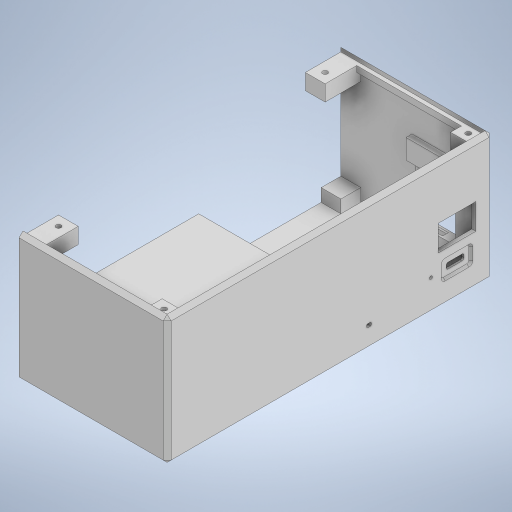
# Autodesk Inventor part: base
Saved by Autodesk Inventor 2024.2 (Build 282272000, 272)
## iProperties
Created: 2024-05-15
Part Number: base
Material: Générique
Document SubType Name: Modeling
Designer: michgae
Density: 1 g/cm^3
Appearance: Par défaut
Author: michgae
Autodesk Inventor part; units mm, degrees
ref_plane "YZ Plane" through (0, 0, 0) normal (1, 0, 0) x (0, 1, 0)
ref_plane "XZ Plane" through (0, 0, 0) normal (0, 1, 0) x (-1, 0, 0)
ref_plane "XY Plane" through (0, 0, 0) normal (0, 0, 1) x (1, 0, 0)
sketch "Esquisse1" plane through (0, 0, 0) normal (0, 0, 1) x (1, 0, 0)
  line L0 (37.5, -32.5) -> (-37.5, -32.5)
  line L1 (-37.5, -32.5) -> (-37.5, 32.5)
  line L2 (-37.5, 32.5) -> (37.5, 32.5)
  line L3 (37.5, 32.5) -> (37.5, -32.5)
  line L4 (0, -45.5) -> (0, 45.5) projected
  line L5 (-52.5, 0) -> (52.5, 0) projected
  line L6 (-37.5, -30.5) -> (35.5, -30.5)
  line L7 (35.5, -30.5) -> (35.5, 32.5)
  point P0 (0, 0)
  dimension "d0" = 75
  dimension "d1" = 65
  dimension "d2" = 32.5
  dimension "d3" = 2
  dimension "d4" = 2
  constraints: 12 end point, 2 horizontal, 2 parallel, 2 perpendicular, 2 point on line, 1 other
  measures "d0" distance of L2.end L1.end
  measures "d1" distance of L1.end L0.end
  measures "d2" distance between parallel lines of L5 L0
  measures "d3" distance between parallel lines of L3 L7
  measures "d4" distance between parallel lines of L0 L6
extrude "Extrusion1" add sketch "Esquisse1" along normal blind 2
extrude "Extrusion2" add sketch "Esquisse1" against normal blind 161 contours L0 L4 L6 L7 L5 L3 | L0 L1 L6 L4 | L5 L7 L2 L3
sketch "Esquisse4" plane through (0, 0, -161) normal (0, 0, -1) x (-1, 0, 0)
  line L0 (37.5, 32.5) -> (37.5, -32.5) projected
  line L1 (-37.5, -32.5) -> (37.5, -32.5)
  line L2 (37.5, -32.5) -> (37.5, 32.5)
  line L3 (37.5, 32.5) -> (-37.5, 32.5)
  line L4 (-37.5, 32.5) -> (-37.5, -32.5)
  point P0 (0, 0)
  constraints: 8 end point, 2 parallel, 1 horizontal, 1 perpendicular
extrude "Extrusion5" add sketch "Esquisse4" along normal blind 2
sketch "Esquisse7" plane through (-37.5, -30.5, 0) normal (0, 1, 0) x (1, 0, 0)
  circle A0 centre (69.5, 152.5) radius 1
  line L0 (73, 0) -> (73, 161) projected
  line L1 (0, 161) -> (73, 161) projected
  circle A1 centre (68.5, 9.5) radius 1
  line L2 (73, 0) -> (0, 0) projected
  line L3 (73, 161) -> (63, 161)
  line L4 (63, 161) -> (63, 146)
  line L5 (63, 146) -> (73, 146)
  line L6 (73, 146) -> (73, 161)
  line L7 (73, 0) -> (63, 0)
  line L8 (63, 0) -> (63, 15)
  line L9 (63, 15) -> (73, 15)
  line L10 (73, 15) -> (73, 0)
  point P0 (37.5, 0)
  point P1 (63, 0)
  dimension "d32" = 2
  dimension "d33" = 3.5
  dimension "d34" = 8.5
  dimension "d35" = 2
  dimension "d36" = 4.5
  dimension "d37" = 9.5
  dimension "d38" = 10
  dimension "d39" = 15
  dimension "d40" = 15
  dimension "d41" = 10
  constraints: 16 end point, 4 parallel, 2 centre point, 2 horizontal, 2 perpendicular
  measures "d32" diameter of A0
  measures "d33" distance from line of L0 A0.centre
  measures "d34" distance from line of L1 A0.centre
  measures "d35" diameter of A1
  measures "d36" distance from line of L0 A1.centre
  measures "d37" distance from line of L2 A1.centre
  measures "d38" distance of L5.end L4.end
  measures "d39" distance of L4.end L3.end
  measures "d40" distance of L7.end L8.end
  measures "d41" distance of L8.end L9.end
extrude "Extrusion7" add sketch "Esquisse7" along normal blind 6.5
sketch "Esquisse8" plane through (35.5, 32.5, -161) normal (-1, 0, 0) x (0, 0, 1)
  line L0 (12.7, -50.3) -> (19.7, -50.3)
  line L1 (20.7, -49.3) -> (20.7, -48.3)
  line L2 (19.7, -47.3) -> (12.7, -47.3)
  line L3 (11.7, -48.3) -> (11.7, -49.3)
  line L4 (0, -56.5) -> (15, -56.5) projected
  line L5 (10.2, -44.8) -> (22.2, -44.8)
  line L6 (23.2, -45.8) -> (23.2, -51.8)
  line L7 (22.2, -52.8) -> (10.2, -52.8)
  line L8 (9.2, -51.8) -> (9.2, -45.8)
  line L9 (0, -63) -> (0, 0) projected
  arc A0 (12.7, -47.3) -> (11.7, -48.3) centre (12.7, -48.3) ccw
  arc A1 (11.7, -49.3) -> (12.7, -50.3) centre (12.7, -49.3) ccw
  arc A2 (19.7, -50.3) -> (20.7, -49.3) centre (19.7, -49.3) ccw
  arc A3 (20.7, -48.3) -> (19.7, -47.3) centre (19.7, -48.3) ccw
  arc A4 (10.2, -44.8) -> (9.2, -45.8) centre (10.2, -45.8) ccw
  arc A5 (23.2, -45.8) -> (22.2, -44.8) centre (22.2, -45.8) ccw
  arc A6 (22.2, -52.8) -> (23.2, -51.8) centre (22.2, -51.8) ccw
  arc A7 (9.2, -51.8) -> (10.2, -52.8) centre (10.2, -51.8) ccw
  circle A8 centre (29.45, -48.8) radius 0.75
  circle A9 centre (60.8, -53.85) radius 1.25
  line L10 (59.9, -52.9825) -> (61.7, -52.9825)
  line L11 (59.9, -54.7175) -> (61.7, -54.7175)
  line L12 (6.7, -39.8) -> (25.7, -39.8)
  line L13 (25.7, -39.8) -> (25.7, -26.8)
  line L14 (25.7, -26.8) -> (6.7, -26.8)
  line L15 (6.7, -26.8) -> (6.7, -39.8)
  point P0 (161, -32.5)
  point P1 (11.7, -50.3)
  point P2 (20.7, -47.3)
  point P3 (11.7, -47.3)
  point P4 (9.2, -44.8)
  point P5 (23.2, -52.8)
  point P6 (23.2, -44.8)
  point P7 (16.2, -52.8)
  dimension "d44" = 6.2
  dimension "d45" = 3
  dimension "d46" = 8
  dimension "d47" = 14
  dimension "d48" = 9
  dimension "d49" = 2.5
  dimension "d50" = 11.7
  dimension "d52" = 1
  dimension "d57" = 9.2
  dimension "d58" = 1.5
  dimension "d59" = 6.25
  dimension "d60" = 4
  dimension "d63" = 2.5
  dimension "d64" = 60.8
  dimension "d65" = 2.65
  dimension "d68" = 1.8
  dimension "d69" = 1.8
  dimension "d70" = 19
  dimension "d71" = 13
  dimension "d72" = 2.5
  dimension "d73" = 5
  constraints: 28 end point, 20 point on circle, 16 tangent, 12 point on line, 10 centre point, 7 equal radius, 6 parallel, 5 horizontal, 3 perpendicular, 1 midpoint
  measures "d44" distance between parallel lines of L0 L4
  measures "d45" distance of point (11.7, -47.3) point (11.7, -50.3)
  measures "d46" distance of point (23.2, -44.8) point (23.2, -52.8)
  measures "d47" distance of point (9.2, -44.8) point (23.2, -44.8)
  measures "d48" distance of point (20.7, -47.3) point (11.7, -47.3)
  measures "d49" distance from line of point (16.2, -52.8) L0
  measures "d50" distance between parallel lines of L3 L9
  measures "d52" radius of A0
  measures "d57" distance between parallel lines of L9 L8
  measures "d58" diameter of A8
  measures "d59" distance from line of L6 A8.centre
  measures "d60" distance from line of L7 A8.centre
  measures "d63" diameter of A9
  measures "d64" distance from line of L9 A9.centre
  measures "d65" distance from line of L4 A9.centre
  measures "d68" distance of L10.start L10.end
  measures "d69" distance of L11.start L11.end
  measures "d70" distance of L14.end L13.end
  measures "d71" distance of L13.end L12.end
  measures "d72" distance between parallel lines of L6 L13
  measures "d73" distance between parallel lines of L12 L5
extrude "Extrusion8" cut sketch "Esquisse8" against normal through all contours A1 L3 A0 L2 A3 L1 A2 L0 | L5 A5 L6 A6 L7 A7 L8 A4
extrude "Extrusion9" add sketch "Esquisse8" against normal blind 1 contours L5 A5 L6 A6 L7 A7 L8 A4
extrude "Extrusion10" cut sketch "Esquisse8" against normal through all contours A8
extrude "Extrusion11" cut sketch "Esquisse8" against normal through all contours A9 L11 L10
extrude "Extrusion12" cut sketch "Esquisse8" against normal through all contours L15 L14 L13 L12
sketch "Esquisse9" plane through (0, 0, -161) normal (0, 0, 1) x (1, 0, 0)
  line L0 (0.5, -22.5) -> (20.5, -22.5)
  line L1 (20.5, -22.5) -> (20.5, 7.5)
  line L2 (20.5, 7.5) -> (0.5, 7.5)
  line L3 (0.5, 7.5) -> (0.5, -22.5)
  line L4 (35.5, -24) -> (35.5, 32.5) projected
  line L5 (-37.5, -30.5) -> (25.5, -30.5) projected
  line L6 (-1.5, 12.5) -> (22.5, 12.5)
  line L7 (22.5, 12.5) -> (22.5, 2.5)
  line L8 (22.5, 2.5) -> (-1.5, 2.5)
  line L9 (-1.5, 2.5) -> (-1.5, 12.5)
  circle A0 centre (10.5, 5) radius 1.25
  line L10 (23, -22.5) -> (-2, -22.5)
  line L11 (-2, -22.5) -> (-2, -27.5)
  line L12 (-2, -27.5) -> (23, -27.5)
  line L13 (23, -27.5) -> (23, -22.5)
  line L14 (-37.5, 32.5) -> (-27.5, 32.5)
  line L15 (-27.5, 32.5) -> (-27.5, 22.5)
  line L16 (-27.5, 22.5) -> (-37.5, 22.5)
  line L17 (-37.5, 22.5) -> (-37.5, 32.5)
  line L18 (-37.5, -30.5) -> (-27.5, -30.5)
  line L19 (-27.5, -30.5) -> (-27.5, -24)
  line L20 (-27.5, -24) -> (-37.5, -24)
  line L21 (-37.5, -24) -> (-37.5, -30.5)
  point P0 (0, 0)
  point P1 (22.5, 7.5)
  point P2 (-1.5, 7.5)
  point P3 (23, -25)
  dimension "d77" = 35
  dimension "d78" = 20
  dimension "d79" = 8
  dimension "d80" = 30
  dimension "d81" = 2
  dimension "d82" = 2
  dimension "d83" = 5
  dimension "d84" = 10
  dimension "d85" = 2.5
  dimension "d86" = 2.5
  dimension "d87" = 10
  dimension "d88" = 25
  dimension "d89" = 2.5
  dimension "d90" = 5
  dimension "d104" = 10
  dimension "d105" = 10
  dimension "d113" = 10
  dimension "d114" = 6.5
  constraints: 40 end point, 10 parallel, 5 horizontal, 5 perpendicular, 3 midpoint, 1 centre point, 1 collinear
  measures "d77" distance between parallel lines of L4 L3
  measures "d78" distance of L1.end L2.end
  measures "d79" distance between parallel lines of L0 L5
  measures "d80" distance of L2.end L0.start
  measures "d81" distance from line of point (22.5, 7.5) L1
  measures "d82" distance from line of L3 point (-1.5, 7.5)
  measures "d83" distance between parallel lines of L2 L6
  measures "d84" distance between parallel lines of L6 L8
  measures "d85" diameter of A0
  measures "d86" distance from line of L2 A0.centre
  measures "d87" distance from line of L1 A0.centre
  measures "d88" distance of L12.end L11.end
  measures "d89" distance from line of L1 point (23, -25)
  measures "d90" distance of L10.end L11.end
  measures "d104" distance of L15.end L16.end
  measures "d105" distance of L14.end L15.end
  measures "d113" distance of L20.end L19.end
  measures "d114" distance of L19.end L18.end
extrude "Extrusion13" cut sketch "Esquisse9" against normal blind 10 contours L3 L8 L1 L0 | L3 L2 L1 L8 | A0
extrude "Extrusion14" add sketch "Esquisse9" along normal blind 3 contours L0 L10 L13 L12 L11 | L8 L9 L6 L7 L1 L2 L3 | L3 L2 L1 L8
sketch "Esquisse10" plane through (0.5, -22.5, -163) normal (0, 1, 0) x (1, 0, 0)
  line L0 (15, -1.5) -> (5, -1.5)
  line L1 (5, -1.5) -> (5, -3.5)
  line L2 (5, -3.5) -> (15, -3.5)
  line L3 (15, -3.5) -> (15, -1.5)
  line L4 (0, 0) -> (20, 0) projected
  line L5 (20, -2) -> (20, 0) projected
  point P0 (-0.5, -163)
  dimension "d95" = 10
  dimension "d96" = 2
  dimension "d97" = 1.5
  dimension "d98" = 5
  constraints: 8 end point, 2 parallel, 1 horizontal, 1 perpendicular
  measures "d95" distance of L1.end L2.end
  measures "d96" distance of L0.end L1.end
  measures "d97" distance between parallel lines of L4 L0
  measures "d98" distance between parallel lines of L5 L3
extrude "Extrusion15" cut sketch "Esquisse10" against normal blind 3
chamfer "Chanfrein1" distance 0.5 angle 45 4 edges at (15.5, -22.5, -160.5) (10.5, -22.5, -159.5) (10.5, -22.5, -161.5) (5.5, -22.5, -160.5)
extrude "Extrusion16" add sketch "Esquisse9" along normal blind 18 contours L14 L15 L16 L17
extrude "Extrusion18" add sketch "Esquisse9" along normal blind 10 contours L21 L20 L19 L5
sketch "Esquisse12" plane through (0, 0, 0) normal (0, 0, -1) x (-1, 0, 0)
  line L0 (-25.5, -30.5) -> (37.5, -30.5) projected
  line L1 (37.5, -30.5) -> (27.5, -30.5)
  line L2 (27.5, -30.5) -> (27.5, -24)
  line L3 (27.5, -24) -> (37.5, -24)
  line L4 (37.5, -24) -> (37.5, -30.5)
  line L5 (37.5, 32.5) -> (37.5, -32.5) projected
  line L6 (37.5, 32.5) -> (27.5, 32.5)
  line L7 (27.5, 32.5) -> (27.5, 22.5)
  line L8 (27.5, 22.5) -> (37.5, 22.5)
  line L9 (37.5, 22.5) -> (37.5, 32.5)
  point P0 (0, 0)
  dimension "d120" = 10
  dimension "d121" = 6.5
  dimension "d122" = 10
  dimension "d123" = 10
  constraints: 16 end point, 4 parallel, 2 horizontal, 2 perpendicular
  measures "d120" distance of L2.end L3.end
  measures "d121" distance of L1.end L2.end
  measures "d122" distance of L8.end L7.end
  measures "d123" distance of L7.end L6.end
extrude "Extrusion19" add sketch "Esquisse12" along normal blind 18 contours L5 L8 L7 L6
extrude "Extrusion20" add sketch "Esquisse12" along normal blind 10 contours L2 L3 L4 L0
sketch "Esquisse11" plane through (-37.5, -32.5, 2) normal (-1, 0, 0) x (0, 0, 1)
  circle A0 centre (-160, 60) radius 1.25
  line L0 (-145, 65) -> (-165, 65) projected
  line L1 (-165, 0) -> (-165, 65) projected
  circle A1 centre (-160, 5) radius 1.25
  line L2 (-165, 0) -> (0, 0) projected
  circle A2 centre (-5, 60) radius 1.25
  circle A3 centre (-5, 5) radius 1.25
  point P0 (-2, 32.5)
  dimension "d108" = 2.5
  dimension "d109" = 5
  dimension "d110" = 5
  dimension "d117" = 2.5
  dimension "d118" = 5
  dimension "d119" = 5
  dimension "d130" = 155
  constraints: 4 centre point, 1 horizontal, 4 other
  measures "d108" diameter of A0
  measures "d109" distance from line of L0 A0.centre
  measures "d110" distance from line of L1 A0.centre
  measures "d117" diameter of A1
  measures "d118" distance from line of L2 A1.centre
  measures "d119" distance from line of L1 A1.centre
  measures "d130" distance of A0.centre A2.centre
extrude "Extrusion17" cut sketch "Esquisse11" against normal blind 9
sketch "Esquisse13" plane through (35.5, 32.5, -161) normal (-1, 0, 0) x (0, 0, 1)
  line L0 (161, 0) -> (0, 0) projected
  line L1 (0, 0) -> (7.5, 0)
  line L2 (7.5, 0) -> (7.5, -10)
  line L3 (7.5, -10) -> (0, -10)
  line L4 (0, -10) -> (0, 0)
  line L5 (0, -56.5) -> (0, 0) projected
  line L6 (161, 0) -> (153.5, 0)
  line L7 (153.5, 0) -> (153.5, -10)
  line L8 (153.5, -10) -> (161, -10)
  line L9 (161, -10) -> (161, 0)
  line L10 (0, -2) -> (161, -2)
  line L11 (161, -2) -> (161, -5)
  line L12 (161, -5) -> (0, -5)
  line L13 (0, -5) -> (0, -2)
  line L14 (2, -2) -> (2, -5)
  line L15 (159, -2) -> (159, -5)
  point P0 (161, -32.5)
  point P1 (7.5, 0)
  point P2 (0, -3.5)
  point P3 (2, -3.5)
  point P4 (161, -3.5)
  point P5 (0, -5)
  point P6 (161, -2)
  dimension "d135" = 7.5
  dimension "d136" = 10
  dimension "d137" = 0
  dimension "d138" = 7.5
  dimension "d139" = 10
  dimension "d167" = 3
  dimension "d168" = 2
  dimension "d169" = 2
  dimension "d170" = 2
  constraints: 28 end point, 6 parallel, 6 point on line, 5 perpendicular, 4 midpoint, 3 horizontal
  measures "d135" distance of L2.end L3.end
  measures "d136" distance of L1.end L2.end
  measures "d137" distance between parallel lines of L5 L4
  measures "d138" distance of L8.end L7.end
  measures "d139" distance of L7.end L6.end
  measures "d167" distance of L10.end L11.end
  measures "d168" distance between parallel lines of L10 L0
  measures "d169" distance of point (0, -3.5) point (2, -3.5)
  measures "d170" distance from line of point (161, -3.5) L15
extrude "Extrusion21" add sketch "Esquisse13" along normal blind 10 contours L9 L10 L7 L0 | L9 L12 L15 L10 | L2 L10 L4 L0 | L10 L15 L12 L7 | L9 L8 L7 L12 | L2 L12 L14 L10 | L10 L14 L12 L4 | L2 L3 L4 L12
sketch "Esquisse14" plane through (-37.5, 32.5, 2) normal (0, 1, 0) x (1, 0, 0)
  circle A0 centre (68, 159.5) radius 1.25
  line L0 (75, 165) -> (75, 0) projected
  line L1 (0, 165) -> (75, 165) projected
  circle A1 centre (68, 5.5) radius 1.25
  circle A2 centre (5, 150) radius 1.25
  line L2 (10, 163) -> (10, 145) projected
  line L3 (10, 145) -> (0, 145) projected
  circle A3 centre (5, 15) radius 1.25
  point P0 (37.5, 2)
  dimension "d142" = 2.5
  dimension "d143" = 7
  dimension "d144" = 5.5
  dimension "d147" = 154
  dimension "d152" = 2.5
  dimension "d153" = 5
  dimension "d154" = 5
  dimension "d157" = 135
  constraints: 4 centre point, 2 vertical, 4 other
  measures "d142" diameter of A0
  measures "d143" distance from line of L0 A0.centre
  measures "d144" distance from line of L1 A0.centre
  measures "d147" distance of A0.centre A1.centre
  measures "d152" diameter of A2
  measures "d153" distance from line of L2 A2.centre
  measures "d154" distance from line of L3 A2.centre
  measures "d157" distance of A2.centre A3.centre
extrude "Extrusion22" cut sketch "Esquisse14" against normal blind 9
chamfer "Chanfrein2" distance 2 angle 45 8 edges at (0, 32.5, -163) (37.5, 0, -163) (37.5, 32.5, -80.5) (0, -32.5, -163) (37.5, -32.5, -80.5) (0, -32.5, 2) (37.5, 0, 2) (0, 32.5, 2)
extrude "Extrusion23" add sketch "Esquisse13" along normal blind 65 contours L9 L12 L15 L10 | L10 L14 L12 L4
extrude "Extrusion24" add sketch "Esquisse13" along normal blind 2 contours L10 L15 L12 L7 | L7 L12 L2 L10 | L2 L12 L14 L10
extrude "Extrusion25" cut sketch "Esquisse13" along normal through all contours L9 L10 L7 L0 | L7 L10 L2 L0 | L2 L10 L4 L0
sketch "Esquisse16" plane through (0, 0, 0) normal (0, 0, -1) x (-1, 0, 0)
  line L0 (-18.5, 11.5) -> (21.5, 11.5)
  line L1 (21.5, 11.5) -> (21.5, 9.5)
  line L2 (21.5, 9.5) -> (-18.5, 9.5)
  line L3 (-18.5, 9.5) -> (-18.5, 11.5)
  line L4 (-25.5, -30.5) -> (27.5, -30.5) projected
  line L5 (37.5, 22.5) -> (37.5, -24) projected
  point P0 (0, 0)
  point P1 (21.5, 10.5)
  dimension "d177" = 42
  dimension "d178" = 2
  dimension "d179" = 16
  dimension "d180" = 40
  constraints: 8 end point, 2 parallel, 1 horizontal, 1 midpoint, 1 perpendicular
  measures "d177" distance between parallel lines of L4 L0
  measures "d178" distance of L0.end L1.end
  measures "d179" distance from line of L5 point (21.5, 10.5)
  measures "d180" distance of L0.start L0.end
extrude "Extrusion26" add sketch "Esquisse16" along normal blind 75
sketch "Esquisse17" plane through (18.5, 9.5, 0) normal (1, 0, 0) x (0, 0, -1)
  line L0 (75, 0) -> (25, 0)
  line L1 (25, 0) -> (25, 2)
  line L2 (25, 2) -> (75, 2)
  line L3 (75, 2) -> (75, 0)
  point P0 (0, -9.5)
  dimension "d183" = 50
  dimension "d184" = 2
  constraints: 8 end point, 2 parallel, 1 horizontal, 1 perpendicular
  measures "d183" distance of L1.end L2.end
  measures "d184" distance of L0.end L1.end
extrude "Extrusion27" add sketch "Esquisse17" along normal up to surface (17 mm away)
sketch "Esquisse18" plane through (0, 0, -75) normal (0, 0, -1) x (-1, 0, 0)
  line L0 (21.5, 9.5) -> (21.5, 11.5) projected
  line L1 (-35.5, 11.5) -> (-35.5, 9.5) projected
  line L2 (-35.5, 9.5) -> (-35.5, 11.5) projected
  line L3 (-35.5, -17.8) -> (-35.5, -16.8) projected
  line L4 (-35.5, -16.8) -> (-35.5, -15.8) projected
  line L5 (-35.5, -15.8) -> (-35.5, -14.8) projected
  line L6 (-35.5, -14.8) -> (-35.5, -15.8) projected
  line L7 (-35.5, -15.8) -> (-35.5, -16.8) projected
  line L8 (-35.5, -16.8) -> (-35.5, -17.8) projected
  line L9 (-35.5, -15.55) -> (-35.5, -17.05) projected
  line L10 (-35.5, -20.4825) -> (-35.5, -22.2175) projected
  line L11 (-35.5, -22.2175) -> (-35.5, -20.4825) projected
  line L12 (-35.5, 5.7) -> (-35.5, -7.3) projected
  line L13 (-35.5, -7.3) -> (-35.5, 5.7) projected
  line L14 (-35.5, 27.5) -> (-35.5, 22.5) projected
  line L15 (-35.5, -24) -> (-35.5, 22.5) projected
  line L16 (-35.5, -24) -> (-35.5, -30.5) projected
  line L17 (-35.5, -30.5) -> (-35.5, -24) projected
  line L18 (-35.5, 22.5) -> (-35.5, -24) projected
  line L19 (-35.5, 22.5) -> (-35.5, 27.5) projected
  line L20 (21.5, 9.5) -> (-35.5, -15.5)
  line L21 (21.5, 9.5) -> (-18.5, 9.5) projected
  line L22 (21.5, 9.5) -> (-35.5, 9.5) projected
  line L23 (-18.5, 9.5) -> (-35.5, 9.5) projected
  line L24 (21.5, 9.5) -> (16.5, 9.5)
  line L25 (-35.5, -13.307) -> (-35.5, -15.5)
  line L26 (-37.5, -30.5) -> (-37.5, 30.5) projected
  line L27 (16.5, 9.5) -> (-35.5, 9.5)
  line L28 (-35.5, -13.307) -> (-35.5, 9.5)
  point P0 (0, 0)
  point P1 (-35.5, -15.5)
  dimension "d187" = 25
  dimension "d188" = 5
  constraints: 10 end point, 3 point on line, 2 collinear, 1 parallel
  measures "d187" distance of L1.end L20.end
  measures "d188" distance of L0.start L24.end
extrude "Extrusion28" add sketch "Esquisse18" against normal blind 5
chamfer "Chanfrein3" distance 2 angle 45 5 edges at (7, -3, -75) (7, 11.5, -75) (7, -3, -70) (27, 11.5, -25) (18.5, 11.5, -12.5)
chamfer "Chanfrein4" distance 1 angle 45 8 edges at (37.5, -12.3, -144.8) (37.5, -12.5929, -151.5071) (37.5, -16.3, -151.8) (37.5, -20.0071, -151.5071) (37.5, -20.3, -144.8) (37.5, -20.0071, -138.0929) (37.5, -16.3, -137.8) (37.5, -12.5929, -138.0929)
equation "\"d49\" = -0.5 * d45 + 0.5 * d46"
equation "\"d57\" = d50 - 0.5 * d47 + 0.5 * d48"
